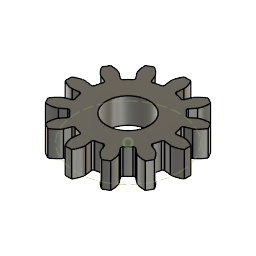
RightLegJoint (Autodesk Fusion 360 archive; units mm, degrees)
design "SmallGear_12Teeth_30mThickness_50mHole"
description: Spur Gear; Module: 10.0; Num Teeth: 12; Pressure Angle: 14.500000000000002; Backlash: 0.00 mm
Autodesk Fusion 360 part; units mm, degrees
sketch "Base Circle" plane through (0, 0, 0) normal (0, 0, 1) x (1, 0, 0)
  circle A0 centre (0, 0) radius 48.43
  circle A1 centre (0, 0) radius 25
extrude "Extrude1" add sketch "Base Circle" along normal blind 30
sketch "Gear Tooth" plane through (0, 0, 0) normal (0, 0, 1) x (1, 0, 0)
  spline S0 degree 5 poles (57.549, -7.9013) (57.5843, -7.9062) (57.655, -7.9148) (57.7612, -7.9246) (57.9033, -7.9318) (58.0814, -7.9325) (58.26, -7.9274) (58.4388, -7.9188) (58.6177, -7.9084) (58.7967, -7.8966) (58.9758, -7.8833) (59.1549, -7.8682) (59.3341, -7.8506) (59.5134, -7.8301) (59.6927, -7.8067) (59.8721, -7.7808) (60.0515, -7.7525) (60.2309, -7.7225) (60.4103, -7.6908) (60.5896, -7.6576) (60.7688, -7.6227) (60.9481, -7.5862) (61.1272, -7.548) (61.3063, -7.508) (61.4854, -7.4662) (61.6643, -7.4227) (61.8432, -7.3776) (62.022, -7.331) (62.2007, -7.283) (62.3792, -7.2335) (62.5577, -7.1826) (62.7361, -7.1302) (62.9143, -7.0764) (63.0924, -7.0212) (63.2703, -6.9646) (63.4482, -6.9066) (63.6258, -6.8473) (63.8034, -6.7866) (63.9808, -6.7246) (64.158, -6.6613) (64.335, -6.5968) (64.5119, -6.531) (64.6886, -6.4639) (64.8652, -6.3956) (65.0415, -6.326) (65.2177, -6.2552) (65.3937, -6.1832) (65.5695, -6.11) (65.7451, -6.0356) (65.9205, -5.9601) (66.0956, -5.8834) (66.2706, -5.8055) (66.4454, -5.7265) (66.6199, -5.6463) (66.7942, -5.565) (66.9683, -5.4826) (67.1422, -5.3991) (67.3159, -5.3145) (67.4893, -5.2288) (67.6624, -5.142) (67.8354, -5.0541) (68.008, -4.9652) (68.1805, -4.8752) (68.3526, -4.7841) (68.5246, -4.692) (68.6962, -4.5988) (68.8676, -4.5047) (69.0388, -4.4095) (69.2096, -4.3132) (69.3802, -4.216) (69.5505, -4.1177) (69.6866, -4.0383) (69.7885, -3.9783) (69.8563, -3.9381) (69.8903, -3.918) knots 0 0 0 0 0 0 0.01428571 0.02857143 0.04285714 0.05714286 0.07142857 0.08571429 0.1 0.11428571 0.12857143 0.14285714 0.15714286 0.17142857 0.18571429 0.2 0.21428571 0.22857143 0.24285714 0.25714286 0.27142857 0.28571429 0.3 0.31428571 0.32857143 0.34285714 0.35714286 0.37142857 0.38571429 0.4 0.41428571 0.42857143 0.44285714 0.45714286 0.47142857 0.48571429 0.5 0.51428571 0.52857143 0.54285714 0.55714286 0.57142857 0.58571429 0.6 0.61428571 0.62857143 0.64285714 0.65714286 0.67142857 0.68571429 0.7 0.71428571 0.72857143 0.74285714 0.75714286 0.77142857 0.78571429 0.8 0.81428571 0.82857143 0.84285714 0.85714286 0.87142857 0.88571429 0.9 0.91428571 0.92857143 0.94285714 0.95714286 0.97142857 0.98571429 1 1 1 1 1 1
  spline S1 degree 5 poles (57.549, 7.9013) (57.5843, 7.9062) (57.655, 7.9148) (57.7612, 7.9246) (57.9033, 7.9318) (58.0814, 7.9325) (58.26, 7.9274) (58.4388, 7.9188) (58.6177, 7.9084) (58.7967, 7.8966) (58.9758, 7.8833) (59.1549, 7.8682) (59.3341, 7.8506) (59.5134, 7.8301) (59.6927, 7.8067) (59.8721, 7.7808) (60.0515, 7.7525) (60.2309, 7.7225) (60.4103, 7.6908) (60.5896, 7.6576) (60.7688, 7.6227) (60.9481, 7.5862) (61.1272, 7.548) (61.3063, 7.508) (61.4854, 7.4662) (61.6643, 7.4227) (61.8432, 7.3776) (62.022, 7.331) (62.2007, 7.283) (62.3792, 7.2335) (62.5577, 7.1826) (62.7361, 7.1302) (62.9143, 7.0764) (63.0924, 7.0212) (63.2703, 6.9646) (63.4482, 6.9066) (63.6258, 6.8473) (63.8034, 6.7866) (63.9808, 6.7246) (64.158, 6.6613) (64.335, 6.5968) (64.5119, 6.531) (64.6886, 6.4639) (64.8652, 6.3956) (65.0415, 6.326) (65.2177, 6.2552) (65.3937, 6.1832) (65.5695, 6.11) (65.7451, 6.0356) (65.9205, 5.9601) (66.0956, 5.8834) (66.2706, 5.8055) (66.4454, 5.7265) (66.6199, 5.6463) (66.7942, 5.565) (66.9683, 5.4826) (67.1422, 5.3991) (67.3159, 5.3145) (67.4893, 5.2288) (67.6624, 5.142) (67.8354, 5.0541) (68.008, 4.9652) (68.1805, 4.8752) (68.3526, 4.7841) (68.5246, 4.692) (68.6962, 4.5988) (68.8676, 4.5047) (69.0388, 4.4095) (69.2096, 4.3132) (69.3802, 4.216) (69.5505, 4.1177) (69.6866, 4.0383) (69.7885, 3.9783) (69.8563, 3.9381) (69.8903, 3.918) knots 0 0 0 0 0 0 0.01428571 0.02857143 0.04285714 0.05714286 0.07142857 0.08571429 0.1 0.11428571 0.12857143 0.14285714 0.15714286 0.17142857 0.18571429 0.2 0.21428571 0.22857143 0.24285714 0.25714286 0.27142857 0.28571429 0.3 0.31428571 0.32857143 0.34285714 0.35714286 0.37142857 0.38571429 0.4 0.41428571 0.42857143 0.44285714 0.45714286 0.47142857 0.48571429 0.5 0.51428571 0.52857143 0.54285714 0.55714286 0.57142857 0.58571429 0.6 0.61428571 0.62857143 0.64285714 0.65714286 0.67142857 0.68571429 0.7 0.71428571 0.72857143 0.74285714 0.75714286 0.77142857 0.78571429 0.8 0.81428571 0.82857143 0.84285714 0.85714286 0.87142857 0.88571429 0.9 0.91428571 0.92857143 0.94285714 0.95714286 0.97142857 0.98571429 1 1 1 1 1 1
  arc A0 (69.8903, -3.918) -> (69.8903, 3.918) centre (0, 0) ccw
  line L0 (47.97, -6.5862) -> (57.549, -7.9013)
  line L1 (47.97, 6.5862) -> (57.549, 7.9013)
  line L2 (47.97, -6.5862) -> (47.97, 6.5862)
  point P0 (58.4051, -7.9201)
  point P1 (59.2721, -7.8563)
  point P2 (60.1457, -7.7365)
  point P3 (61.0243, -7.5697)
  point P4 (61.9068, -7.3609)
  point P5 (62.792, -7.1131)
  point P6 (63.6793, -6.8288)
  point P7 (64.5679, -6.5095)
  point P8 (65.4571, -6.1566)
  point P9 (66.3463, -5.7711)
  point P10 (67.2348, -5.3538)
  point P11 (68.122, -4.9055)
  point P12 (69.0074, -4.4267)
  point P13 (58.4051, 7.9201)
  point P14 (59.2721, 7.8563)
  point P15 (60.1457, 7.7365)
  point P16 (61.0243, 7.5697)
  point P17 (61.9068, 7.3609)
  point P18 (62.792, 7.1131)
  point P19 (63.6793, 6.8288)
  point P20 (64.5679, 6.5095)
  point P21 (65.4571, 6.1566)
  point P22 (66.3463, 5.7711)
  point P23 (67.2348, 5.3538)
  point P24 (68.122, 4.9055)
  point P25 (69.0074, 4.4267)
extrude "Extrude2" add sketch "Gear Tooth" along normal blind 30
fillet "Fillet1" radius 2 2 edges at (47.9799, -6.5875, 15) (47.9799, 6.5875, 15)
pattern_circular "C-Pattern1" count 12 over 360 about axis through (0, 0, 0) along (0, 0, 1) of "Extrude2", "Fillet1"
sketch "Diametrial Pitch Circle" plane through (0, 0, 0) normal (0, 0, 1) x (1, 0, 0)
  circle A0 centre (0, 0) radius 60 construction
named bodies: "Spur Gear (12 teeth)"

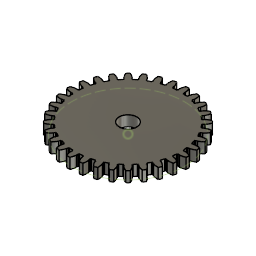
design "BigGear_32Teeth_30mThickness_50mHole"
description: Spur Gear; Module: 10.0; Num Teeth: 32; Pressure Angle: 14.500000000000002; Backlash: 0.00 mm
Autodesk Fusion 360 part; units mm, degrees
sketch "Base Circle" plane through (0, 0, 0) normal (0, 0, 1) x (1, 0, 0)
  circle A0 centre (0, 0) radius 148.43
  circle A1 centre (0, 0) radius 25
extrude "Extrude1" add sketch "Base Circle" along normal blind 30
sketch "Gear Tooth" plane through (0, 0, 0) normal (0, 0, 1) x (1, 0, 0)
  spline S0 degree 5 poles (154.6725, -8.4585) (154.7166, -8.4609) (154.8047, -8.4649) (154.937, -8.4681) (155.1134, -8.4675) (155.3339, -8.4597) (155.5544, -8.447) (155.775, -8.4312) (155.9956, -8.4138) (156.2162, -8.3952) (156.4368, -8.3756) (156.6574, -8.3544) (156.8779, -8.3312) (157.0983, -8.3057) (157.3188, -8.2778) (157.5391, -8.2477) (157.7594, -8.2157) (157.9797, -8.1821) (158.1999, -8.1472) (158.42, -8.111) (158.64, -8.0735) (158.86, -8.0347) (159.0799, -7.9945) (159.2997, -7.9529) (159.5195, -7.9098) (159.7391, -7.8653) (159.9587, -7.8196) (160.1782, -7.7726) (160.3976, -7.7244) (160.6168, -7.675) (160.836, -7.6245) (161.0551, -7.5729) (161.2742, -7.5201) (161.4931, -7.4662) (161.7119, -7.4112) (161.9306, -7.355) (162.1492, -7.2978) (162.3677, -7.2395) (162.586, -7.1801) (162.8043, -7.1198) (163.0225, -7.0584) (163.2405, -6.996) (163.4585, -6.9326) (163.6763, -6.8682) (163.894, -6.8029) (164.1116, -6.7365) (164.329, -6.6693) (164.5464, -6.601) (164.7636, -6.5319) (164.9807, -6.4618) (165.1977, -6.3908) (165.4145, -6.3189) (165.6313, -6.2461) (165.8479, -6.1723) (166.0643, -6.0978) (166.2807, -6.0223) (166.4969, -5.9459) (166.713, -5.8687) (166.9289, -5.7907) (167.1447, -5.7118) (167.3604, -5.632) (167.5759, -5.5514) (167.7913, -5.47) (168.0066, -5.3878) (168.2217, -5.3047) (168.4367, -5.2208) (168.6515, -5.1361) (168.8662, -5.0507) (169.0807, -4.9644) (169.2951, -4.8773) (169.5094, -4.7895) (169.6807, -4.7185) (169.8091, -4.665) (169.8947, -4.6292) (169.9374, -4.6112) knots 0 0 0 0 0 0 0.01428571 0.02857143 0.04285714 0.05714286 0.07142857 0.08571429 0.1 0.11428571 0.12857143 0.14285714 0.15714286 0.17142857 0.18571429 0.2 0.21428571 0.22857143 0.24285714 0.25714286 0.27142857 0.28571429 0.3 0.31428571 0.32857143 0.34285714 0.35714286 0.37142857 0.38571429 0.4 0.41428571 0.42857143 0.44285714 0.45714286 0.47142857 0.48571429 0.5 0.51428571 0.52857143 0.54285714 0.55714286 0.57142857 0.58571429 0.6 0.61428571 0.62857143 0.64285714 0.65714286 0.67142857 0.68571429 0.7 0.71428571 0.72857143 0.74285714 0.75714286 0.77142857 0.78571429 0.8 0.81428571 0.82857143 0.84285714 0.85714286 0.87142857 0.88571429 0.9 0.91428571 0.92857143 0.94285714 0.95714286 0.97142857 0.98571429 1 1 1 1 1 1
  spline S1 degree 5 poles (154.6725, 8.4585) (154.7166, 8.4609) (154.8047, 8.4649) (154.937, 8.4681) (155.1134, 8.4675) (155.3339, 8.4597) (155.5544, 8.447) (155.775, 8.4312) (155.9956, 8.4138) (156.2162, 8.3952) (156.4368, 8.3756) (156.6574, 8.3544) (156.8779, 8.3312) (157.0983, 8.3057) (157.3188, 8.2778) (157.5391, 8.2477) (157.7594, 8.2157) (157.9797, 8.1821) (158.1999, 8.1472) (158.42, 8.111) (158.64, 8.0735) (158.86, 8.0347) (159.0799, 7.9945) (159.2997, 7.9529) (159.5195, 7.9098) (159.7391, 7.8653) (159.9587, 7.8196) (160.1782, 7.7726) (160.3976, 7.7244) (160.6168, 7.675) (160.836, 7.6245) (161.0551, 7.5729) (161.2742, 7.5201) (161.4931, 7.4662) (161.7119, 7.4112) (161.9306, 7.355) (162.1492, 7.2978) (162.3677, 7.2395) (162.586, 7.1801) (162.8043, 7.1198) (163.0225, 7.0584) (163.2405, 6.996) (163.4585, 6.9326) (163.6763, 6.8682) (163.894, 6.8029) (164.1116, 6.7365) (164.329, 6.6693) (164.5464, 6.601) (164.7636, 6.5319) (164.9807, 6.4618) (165.1977, 6.3908) (165.4145, 6.3189) (165.6313, 6.2461) (165.8479, 6.1723) (166.0643, 6.0978) (166.2807, 6.0223) (166.4969, 5.9459) (166.713, 5.8687) (166.9289, 5.7907) (167.1447, 5.7118) (167.3604, 5.632) (167.5759, 5.5514) (167.7913, 5.47) (168.0066, 5.3878) (168.2217, 5.3047) (168.4367, 5.2208) (168.6515, 5.1361) (168.8662, 5.0507) (169.0807, 4.9644) (169.2951, 4.8773) (169.5094, 4.7895) (169.6807, 4.7185) (169.8091, 4.665) (169.8947, 4.6292) (169.9374, 4.6112) knots 0 0 0 0 0 0 0.01428571 0.02857143 0.04285714 0.05714286 0.07142857 0.08571429 0.1 0.11428571 0.12857143 0.14285714 0.15714286 0.17142857 0.18571429 0.2 0.21428571 0.22857143 0.24285714 0.25714286 0.27142857 0.28571429 0.3 0.31428571 0.32857143 0.34285714 0.35714286 0.37142857 0.38571429 0.4 0.41428571 0.42857143 0.44285714 0.45714286 0.47142857 0.48571429 0.5 0.51428571 0.52857143 0.54285714 0.55714286 0.57142857 0.58571429 0.6 0.61428571 0.62857143 0.64285714 0.65714286 0.67142857 0.68571429 0.7 0.71428571 0.72857143 0.74285714 0.75714286 0.77142857 0.78571429 0.8 0.81428571 0.82857143 0.84285714 0.85714286 0.87142857 0.88571429 0.9 0.91428571 0.92857143 0.94285714 0.95714286 0.97142857 0.98571429 1 1 1 1 1 1
  arc A0 (169.9374, -4.6112) -> (169.9374, 4.6112) centre (0, 0) ccw
  line L0 (148.1986, -8.1045) -> (154.6725, -8.4585)
  line L1 (148.1986, 8.1045) -> (154.6725, 8.4585)
  line L2 (148.1986, -8.1045) -> (148.1986, 8.1045)
  point P0 (155.7538, -8.4324)
  point P1 (156.8389, -8.3349)
  point P2 (157.9263, -8.19)
  point P3 (159.0155, -8.0061)
  point P4 (160.1059, -7.7879)
  point P5 (161.1973, -7.5385)
  point P6 (162.2895, -7.2602)
  point P7 (163.3822, -6.9546)
  point P8 (164.4751, -6.6233)
  point P9 (165.5682, -6.2671)
  point P10 (166.6611, -5.8871)
  point P11 (167.7538, -5.484)
  point P12 (168.8459, -5.0585)
  point P13 (155.7538, 8.4324)
  point P14 (156.8389, 8.3349)
  point P15 (157.9263, 8.19)
  point P16 (159.0155, 8.0061)
  point P17 (160.1059, 7.7879)
  point P18 (161.1973, 7.5385)
  point P19 (162.2895, 7.2602)
  point P20 (163.3822, 6.9546)
  point P21 (164.4751, 6.6233)
  point P22 (165.5682, 6.2671)
  point P23 (166.6611, 5.8871)
  point P24 (167.7538, 5.484)
  point P25 (168.8459, 5.0585)
extrude "Extrude2" add sketch "Gear Tooth" along normal blind 30
fillet "Fillet1" radius 2 2 edges at (148.2085, -8.105, 15) (148.2085, 8.105, 15)
pattern_circular "C-Pattern1" count 32 over 360 about axis through (0, 0, 0) along (0, 0, 1) of "Extrude2", "Fillet1"
sketch "Diametrial Pitch Circle" plane through (0, 0, 0) normal (0, 0, 1) x (1, 0, 0)
  circle A0 centre (0, 0) radius 160 construction
named bodies: "Spur Gear (32 teeth)"

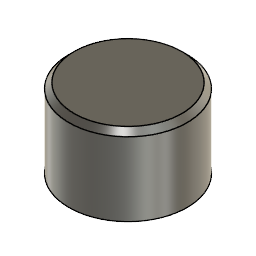
design "Cap"
Autodesk Fusion 360 part; units mm, degrees
sketch "Sketch1" plane through (0, 0, 0) normal (0, 0, 1) x (1, 0, 0)
  circle A0 centre (0, 0) radius 2.25
  line L0 (0, -2.25) -> (0, 2.25) construction
  circle A1 centre (0, 0) radius 2.05
  line L1 (-2.8, 0) -> (3.3, 0) construction
  line L2 (-0.3101, 1.2109) -> (-0.3806, 1.3992)
  line L3 (-0.3101, -1.2109) -> (-0.3806, -1.3992)
  line L4 (0.3101, 1.2109) -> (0.3806, 1.3992)
  line L5 (0.3101, -1.2109) -> (0.3806, -1.3992)
  arc A2 (0.3101, -1.2109) -> (0.3101, 1.2109) centre (0, 0) ccw
  arc A3 (-0.3101, 1.2109) -> (-0.3101, -1.2109) centre (0, 0) ccw
  arc A4 (0.3806, -1.3992) -> (0.3806, 1.3992) centre (0, 0) ccw
  arc A5 (-0.3806, 1.3992) -> (-0.3806, -1.3992) centre (0, 0) ccw
  spline S0 degree 5 poles (-0.6611, 1.2905) (-0.6844, 1.2837) (-0.7307, 1.2707) (-0.7989, 1.2529) (-0.8873, 1.2327) (-0.9934, 1.2139) (-1.0947, 1.2022) (-1.1908, 1.198) (-1.2813, 1.2018) (-1.3665, 1.2133) (-1.4468, 1.2321) (-1.5073, 1.2524) (-1.5508, 1.2704) (-1.5789, 1.2836) (-1.5928, 1.2905) knots 0 0 0 0 0 0 0.1 0.2 0.3 0.4 0.5 0.6 0.7 0.8 0.9 1 1 1 1 1 1
  spline S1 degree 5 poles (-1.1074, 0.936) (-1.124, 0.9409) (-1.1571, 0.9501) (-1.206, 0.9627) (-1.2701, 0.977) (-1.348, 0.9902) (-1.4235, 0.9985) (-1.4965, 1.0014) (-1.5669, 0.9987) (-1.6346, 0.9905) (-1.7, 0.9772) (-1.7506, 0.9629) (-1.7876, 0.9502) (-1.8118, 0.9409) (-1.8238, 0.936) knots 0 0 0 0 0 0 0.1 0.2 0.3 0.4 0.5 0.6 0.7 0.8 0.9 1 1 1 1 1 1
  spline S2 degree 5 poles (-1.1074, -0.936) (-1.124, -0.9409) (-1.1571, -0.9501) (-1.206, -0.9627) (-1.2701, -0.977) (-1.348, -0.9902) (-1.4235, -0.9985) (-1.4965, -1.0014) (-1.5669, -0.9987) (-1.6346, -0.9905) (-1.7, -0.9772) (-1.7506, -0.9629) (-1.7876, -0.9502) (-1.8118, -0.9409) (-1.8238, -0.936) knots 0 0 0 0 0 0 0.1 0.2 0.3 0.4 0.5 0.6 0.7 0.8 0.9 1 1 1 1 1 1
  line L6 (-1.0301, 0.9135) -> (-1.1847, 0.9585)
  line L7 (-1.7583, 0.9626) -> (-1.8894, 0.9095)
  line L8 (-1.0301, -0.9135) -> (-1.1847, -0.9585)
  line L9 (-1.7583, -0.9626) -> (-1.8894, -0.9095)
  spline S3 degree 5 poles (-0.6611, -1.2905) (-0.6844, -1.2837) (-0.7307, -1.2707) (-0.7989, -1.2529) (-0.8873, -1.2327) (-0.9934, -1.2139) (-1.0947, -1.2022) (-1.1908, -1.198) (-1.2813, -1.2018) (-1.3665, -1.2133) (-1.4468, -1.2321) (-1.5073, -1.2524) (-1.5508, -1.2704) (-1.5789, -1.2836) (-1.5928, -1.2905) knots 0 0 0 0 0 0 0.1 0.2 0.3 0.4 0.5 0.6 0.7 0.8 0.9 1 1 1 1 1 1
  line L10 (-0.5569, 1.321) -> (-0.7652, 1.2601)
  line L11 (-1.5135, 1.2509) -> (-1.6721, 1.3301)
  line L12 (-0.5569, -1.321) -> (-0.7652, -1.2601)
  line L13 (-1.5135, -1.2509) -> (-1.6721, -1.3301)
  spline S4 degree 5 poles (0.6611, -1.2905) (0.6844, -1.2837) (0.7307, -1.2707) (0.7989, -1.2529) (0.8873, -1.2327) (0.9934, -1.2139) (1.0947, -1.2022) (1.1908, -1.198) (1.2813, -1.2018) (1.3665, -1.2133) (1.4468, -1.2321) (1.5073, -1.2524) (1.5508, -1.2704) (1.5789, -1.2836) (1.5928, -1.2905) knots 0 0 0 0 0 0 0.1 0.2 0.3 0.4 0.5 0.6 0.7 0.8 0.9 1 1 1 1 1 1
  line L14 (0.5569, -1.321) -> (0.7652, -1.2601)
  line L15 (1.5135, -1.2509) -> (1.6721, -1.3301)
  spline S5 degree 5 poles (1.1074, -0.936) (1.124, -0.9409) (1.1571, -0.9501) (1.206, -0.9627) (1.2701, -0.977) (1.348, -0.9902) (1.4235, -0.9985) (1.4965, -1.0014) (1.5669, -0.9987) (1.6346, -0.9905) (1.7, -0.9772) (1.7506, -0.9629) (1.7876, -0.9502) (1.8118, -0.9409) (1.8238, -0.936) knots 0 0 0 0 0 0 0.1 0.2 0.3 0.4 0.5 0.6 0.7 0.8 0.9 1 1 1 1 1 1
  line L16 (1.0301, -0.9135) -> (1.1847, -0.9585)
  line L17 (1.7583, -0.9626) -> (1.8894, -0.9095)
  spline S6 degree 5 poles (1.1074, 0.936) (1.124, 0.9409) (1.1571, 0.9501) (1.206, 0.9627) (1.2701, 0.977) (1.348, 0.9902) (1.4235, 0.9985) (1.4965, 1.0014) (1.5669, 0.9987) (1.6346, 0.9905) (1.7, 0.9772) (1.7506, 0.9629) (1.7876, 0.9502) (1.8118, 0.9409) (1.8238, 0.936) knots 0 0 0 0 0 0 0.1 0.2 0.3 0.4 0.5 0.6 0.7 0.8 0.9 1 1 1 1 1 1
  line L18 (1.0301, 0.9135) -> (1.1847, 0.9585)
  line L19 (1.7583, 0.9626) -> (1.8894, 0.9095)
  spline S7 degree 5 poles (0.6611, 1.2905) (0.6844, 1.2837) (0.7307, 1.2707) (0.7989, 1.2529) (0.8873, 1.2327) (0.9934, 1.2139) (1.0947, 1.2022) (1.1908, 1.198) (1.2813, 1.2018) (1.3665, 1.2133) (1.4468, 1.2321) (1.5073, 1.2524) (1.5508, 1.2704) (1.5789, 1.2836) (1.5928, 1.2905) knots 0 0 0 0 0 0 0.1 0.2 0.3 0.4 0.5 0.6 0.7 0.8 0.9 1 1 1 1 1 1
  line L20 (0.5569, 1.321) -> (0.7652, 1.2601)
  line L21 (1.5135, 1.2509) -> (1.6721, 1.3301)
  point P0 (-1.2, 1.2)
  point P1 (-1.5, 1)
  point P2 (-1.5, -1)
  point P3 (-1.2, -1.2)
  point P4 (1.2, -1.2)
  point P5 (1.5, -1)
  point P6 (1.5, 1)
  point P7 (1.2, 1.2)
  dimension "d1" = 4.5
  dimension "d2" = 2.5
  dimension "d4" = -0.2
  constraint coincident A0.centre A1.centre
  constraint concentric A0 A2
  constraint coincident A0 L0.start
  constraint coincident A0 L0.end
  constraint vertical L0
  constraint horizontal L1
  constraint symmetric L1 L2.start L3.start
  constraint symmetric L1 L2.end L3.end
  constraint symmetric L0 L2.start L4.start
  constraint symmetric L0 L3.start L5.start
  constraint concentric A2 A4
  constraint concentric A2 A3
  constraint concentric A4 A5
  constraint coincident A5 S0.start
  constraint coincident A1 S0.end
  constraint coincident A5 S1.start
  constraint coincident A1 S1.end
  constraint midpoint S1.start L6
  constraint midpoint S1.end L7
  constraint midpoint S0.start L10
  constraint midpoint S0.end L11
  constraint symmetric L1 S0.start S3.start
  constraint symmetric L1 P0 P3
  constraint symmetric L1 S0.end S3.end
  constraint symmetric L1 S1.start S2.start
  constraint symmetric L1 P1 P2
  constraint symmetric L1 S1.end S2.end
  constraint symmetric L1 L6.start L8.start
  constraint symmetric L1 L6.end L8.end
  constraint symmetric L1 L7.start L9.start
  constraint symmetric L1 L7.end L9.end
  constraint symmetric L1 L10.start L12.start
  constraint symmetric L1 L10.end L12.end
  constraint symmetric L1 L11.start L13.start
  constraint symmetric L1 L11.end L13.end
  constraint symmetric L0 S0.start S7.start
  constraint symmetric L0 P0 P7
  constraint symmetric L0 S0.end S7.end
  constraint symmetric L0 S1.start S6.start
  constraint symmetric L0 P1 P6
  constraint symmetric L0 S1.end S6.end
  constraint symmetric L0 S2.start S5.start
  constraint symmetric L0 P2 P5
  constraint symmetric L0 S2.end S5.end
  constraint symmetric L0 L6.start L18.start
  constraint symmetric L0 L6.end L18.end
  constraint symmetric L0 L7.start L19.start
  constraint symmetric L0 L7.end L19.end
  constraint symmetric L0 L8.start L16.start
  constraint symmetric L0 L8.end L16.end
  constraint symmetric L0 L9.start L17.start
  constraint symmetric L0 L9.end L17.end
  constraint symmetric L0 S3.start S4.start
  constraint symmetric L0 P3 P4
  constraint symmetric L0 S3.end S4.end
  constraint symmetric L0 L10.start L20.start
  constraint symmetric L0 L10.end L20.end
  constraint symmetric L0 L11.start L21.start
  constraint symmetric L0 L11.end L21.end
  constraint symmetric L0 L12.start L14.start
  constraint symmetric L0 L12.end L14.end
  constraint symmetric L0 L13.start L15.start
  constraint symmetric L0 L13.end L15.end
  measures "d1" diameter of A0
  measures "d2" diameter of A2
extrude "Extrude1" add sketch "Sketch1" along normal blind 2 contours A0 | A1 A4 S6 L18 S7 L20 | A1 A5 S0 S1 L6 L10 | L4 L5 A2 A4 | A1 A5 S2 L8 S3 L12 | L2 L3 A3 A5
extrude "Extrude2" add sketch "Sketch1" along normal blind 1 from surface at 2 contours A0 | A1 A4 S5 L16 S6 L18 | A1 A4 S6 L18 S7 L20 | A1 A4 S4 L14 S5 L16 | A1 L2 L3 L4 L5 A2 A3 A4 A5 S0 S3 L10 L12 S4 L14 S7 L20 | A1 A5 S0 S1 L6 L10 | L4 L5 A2 A4 | A1 A5 S2 L8 S3 L12 | A1 A5 S1 S2 L6 L8 | L2 L3 A3 A5
chamfer "Chamfer1" distance 0.2 angle 45 1 edges at (-2.0977, -0.8136, 3)
extrude "Extrude3" add sketch "Sketch1" along normal blind 2 contours A1 A4 S4 S5
